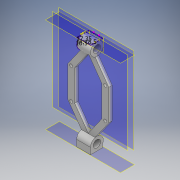
# Autodesk Inventor part: mousetrapMount
Saved by Autodesk Inventor 2018 (Build 220112000, 112)
## iProperties
Created: 2018-11-24
Part Number: mousetrapMount
Material: Generic
Document SubType Name: Modeling
Designer: Prakash
Density: 1 g/cm^3
Appearance: Default
Author: Prakash
Autodesk Inventor part; units mm, degrees
ref_plane "YZ Plane" through (0, 0, 0) normal (1, 0, 0) x (0, 1, 0)
ref_plane "XY Plane" through (0, 0, 0) normal (0, 0, 1) x (1, 0, 0)
sketch "Sketch3" plane through (0, 0, 0) normal (1, 0, 0) x (0, 1, 0)
  circle A0 centre (0, 0) radius 5.25
  circle A1 centre (0, 0) radius 9.25
  dimension "d0" = 10.5
  dimension "d1" = 18.5
  constraints: 2 centre point, 2 coincident
  measures "d0" diameter of A0
  measures "d1" diameter of A1
extrude "Extrusion1" add sketch "Sketch3" along normal blind 20
ref_plane "Work Plane1" through (0, 9.25, 0) normal (0, 1, 0) x (-1, 0, 0)
sketch "Sketch4" plane through (0, 9.25, 0) normal (0, 1, 0) x (-1, 0, 0)
  line L0 (-20, 9.25) -> (-20, -9.25) projected
  line L1 (-20, 0) -> (0, 0) construction
  line L2 (0, 9.25) -> (-20, 9.25) projected
  line L3 (-20, 9.25) -> (-20, -9.25) projected
  line L4 (0, -9.25) -> (0, 9.25) projected
  line L5 (0, -9.25) -> (-20, -9.25) construction
  line L6 (-59.213, -14.8) -> (39.213, -14.8) construction
  line L7 (39.213, -14.8) -> (39.213, -59.25) construction
  line L8 (39.213, -59.25) -> (-59.213, -59.25) construction
  line L9 (-59.213, -59.25) -> (-59.213, -14.8) construction
  line L10 (-59.213, -14.8) -> (39.213, -59.25) construction
  line L11 (39.213, -14.8) -> (-59.213, -59.25) construction
  line L12 (-59.213, -59.25) -> (39.213, -59.25) construction
  line L13 (39.213, -59.25) -> (39.213, -103.7) construction
  line L14 (39.213, -103.7) -> (-59.213, -103.7) construction
  line L15 (-59.213, -103.7) -> (-59.213, -59.25) construction
  line L16 (-59.213, -59.25) -> (39.213, -103.7) construction
  line L17 (39.213, -59.25) -> (-59.213, -103.7) construction
  line L18 (-10, -37.025) -> (-59.213, -37.025) construction
  line L19 (-10, -37.025) -> (39.213, -37.025) construction
  line L20 (-10, -81.475) -> (-59.213, -81.475) construction
  line L21 (-10, -81.475) -> (39.213, -81.475) construction
  line L22 (-20, -9.25) -> (-39.6065, -37.025)
  line L23 (-10, -9.25) -> (-29.6065, -37.025)
  line L24 (-39.6065, -37.025) -> (-39.6065, -59.25)
  line L25 (-10, -9.25) -> (9.6065, -37.025)
  line L26 (0, -9.25) -> (19.6065, -37.025)
  line L27 (19.6065, -37.025) -> (19.6065, -59.25)
  line L28 (-34.6065, -37.025) -> (-34.6065, -81.475) construction
  line L29 (14.6065, -81.475) -> (14.6065, -37.025) construction
  line L30 (-29.6065, -37.025) -> (-29.6065, -59.25)
  line L31 (9.6065, -37.025) -> (9.6065, -59.25)
  line L32 (-39.6065, -59.25) -> (-29.6065, -59.25)
  line L33 (9.6065, -59.25) -> (19.6065, -59.25)
  line L34 (-20, -9.25) -> (-10, -9.25)
  line L35 (0, -9.25) -> (-20, -9.25) projected
  line L36 (-10, -9.25) -> (0, -9.25)
  point P0 (-10, 0)
  dimension "d5" = 44.45
  dimension "d6" = 49.213
  dimension "d7" = 44.45
  dimension "d21" = 50
  constraints: 62 end point, 15 midpoint, 10 point on line, 8 parallel, 5 perpendicular, 3 horizontal, 2 collinear, 2 vertical, 1 equal length, 2 other
  measures "d5" distance of L6.end L7.end
  measures "d6" distance from line of L7 L18.start
  measures "d7" distance of L12.end L13.end
  measures "d21" distance between parallel lines of L8 L5
ref_plane "Work Plane2" through (0, 0, 0) normal (0, 1, 0) x (-1, 0, 0)
sketch "Sketch5" plane through (0, 0, 0) normal (0, 1, 0) x (-1, 0, 0)
  line L0 (-20, -9.25) -> (-39.6065, -37.025) projected
  line L1 (-10, -9.25) -> (-29.6065, -37.025) projected
  line L2 (-10, -9.25) -> (9.6065, -37.025) projected
  line L3 (0, -9.25) -> (19.6065, -37.025) projected
  line L4 (19.6065, -37.025) -> (19.6065, -59.25) projected
  line L5 (9.6065, -37.025) -> (9.6065, -59.25) projected
  line L6 (-29.6065, -37.025) -> (-29.6065, -59.25) projected
  line L7 (-39.6065, -37.025) -> (-39.6065, -59.25) projected
  line L8 (-39.6065, -59.25) -> (-29.6065, -59.25) projected
  line L9 (9.6065, -59.25) -> (19.6065, -59.25) projected
  line L10 (0, -9.25) -> (-20, -9.25) projected
  point P0 (0, 0)
  point P1 (-34.6065, -37.025)
  point P2 (14.6065, -37.025)
extrude "Extrusion2" add sketch "Sketch5" along normal mid plane 5
sketch "Sketch7" plane through (0, -2.5, 0) normal (0, -1, 0) x (1, 0, 0)
  point P0 (0, 0)
  point P1 (34.6065, -37.025)
  point P2 (-14.6065, -37.025)
hole "Hole1" at (-14.6065, -2.5, -37.025) at (34.6065, -2.5, -37.025) direction (0, 1, 0) diameter 4.305 end through all clearance for "Flat Head Machine Screw (82)" size "#6" standard "Ansi Unified Screw Threads"
sketch "Sketch8" plane through (0, 0, -9.25) normal (0, 0, 1) x (-1, 0, 0)
  line L0 (0, -2.5) -> (-10, -2.5) projected
  line L1 (-20, 0) -> (-20, 2.5) projected
  line L2 (0, -2.5) -> (-20, -2.5)
  line L3 (-20, -2.5) -> (-20, 2.5)
  line L4 (-20, 2.5) -> (0, 2.5)
  line L5 (0, 2.5) -> (0, -2.5)
  point P0 (0, 0)
  constraints: 8 end point, 2 parallel, 1 horizontal, 1 perpendicular
extrude "Extrusion4" add sketch "Sketch8" along normal up to surface round surface about axis through (0, 0, 0) along (1, 0, 0) radius 9.25 far side no
ref_plane "Work Plane3" through (0, 0, 9.25) normal (0, 0, -1) x (-1, 0, 0)
ref_plane "Work Plane4" through (0, 0, -127.75) normal (0, 0, -1) x (-1, 0, 0)
ref_plane "Work Plane5" through (0, 9.25, 0) normal (0, 1, 0) x (-1, 0, 0)
sketch "Sketch14" plane through (0, 9.25, 0) normal (0, 1, 0) x (-1, 0, 0)
  line L0 (-20, -8.9058) -> (0, -8.9058) projected
  line L1 (0, -8.9058) -> (0, -8.9058) projected
  line L2 (0, -8.9058) -> (-20, -8.9058) projected
  line L3 (-20, -8.9058) -> (-20, -8.9058) projected
  line L4 (-20, 9.25) -> (-20, -8.9058) projected
  line L5 (0, -8.9058) -> (0, 9.25) projected
  line L6 (-20, -8.9058) -> (0, 9.25) construction
  line L7 (-20, 9.25) -> (0, -8.9058) construction
  point P0 (0, 0)
  point P1 (-10, 0.1721)
  constraints: 4 end point, 1 midpoint
sketch "Sketch15" plane through (0, 9.25, 0) normal (0, 1, 0) x (-1, 0, 0)
  line L0 (-20, 9.25) -> (0, -8.9058) construction
  line L1 (-20, -8.9058) -> (0, 9.25) construction
  circle A0 centre (-10, 0.1721) radius 4
  point P0 (0, 0)
  dimension "d28" = 8
  constraints: 1 centre point, 1 coincident
  measures "d28" diameter of A0
extrude "Extrusion6" add sketch "Sketch15" against normal up to surface round surface about axis through (0, 0, 0) along (1, 0, 0) radius 9.25 far side no
extrude "Extrusion7" add sketch "Sketch15" along normal blind 1
sketch "Sketch16" plane through (10, 10.25, 0.1721) normal (0, 1, 0) x (1, 0, 0)
  line L0 (10, 9.0779) -> (-10, -9.0779) construction
  line L1 (10, -9.0779) -> (-10, 9.0779) construction
  circle A0 centre (0, 0) radius 4 projected
  circle A1 centre (0, 0) radius 2.5275
  point P0 (-10, 0.1721)
  dimension "d33" = 5.055
  constraints: 1 centre point, 1 coincident
  measures "d33" diameter of A1
extrude "Extrusion8" cut sketch "Sketch16" against normal blind 3.81 contours A1
sketch "Sketch17" plane through (10, 10.25, 0.1721) normal (0, 1, 0) x (1, 0, 0)
  line L0 (10, -9.0779) -> (-10, 9.0779) construction
  line L1 (10, 9.0779) -> (-10, -9.0779) construction
  circle A0 centre (0, 0) radius 2.6545
  point P0 (-10, 0.1721)
  dimension "d36" = 5.309
  constraints: 1 centre point, 1 coincident
  measures "d36" diameter of A0
loft "Loft1" cut profiles "Sketch17" section 1 edges at (7.4725, 6.44, 0.1721)
sketch "Sketch18" plane through (10, 6.44, 0.1721) normal (0, 1, 0) x (1, 0, 0)
  line L0 (10, -9.0779) -> (-10, 9.0779) construction
  line L1 (10, 9.0779) -> (-10, -9.0779) construction
  circle A0 centre (0, 0) radius 1.8
  point P0 (-10, 0.1721)
  dimension "d41" = 3.6
  constraints: 1 centre point, 1 coincident
  measures "d41" diameter of A0
extrude "Extrusion9" cut sketch "Sketch18" against normal up to surface round surface about axis through (0, 0, 0) along (1, 0, 0) radius 5.25 far side no
mirror "Mirror3" about plane through (39.6065, 0, -59.25) normal (0, 0, -1) of "Extrusion1", "Extrusion2", "Hole1", "Extrusion4", "Extrusion6", "Extrusion7", "Extrusion8", "Loft1", "Extrusion9"
sketch "Sketch21" plane through (0, 0, 9.25) normal (0, 0, -1) x (-1, 0, 0)
  line L0 (-20, 9.25) -> (-20, -9.25) construction
  line L1 (0, -9.25) -> (0, 9.25) construction
  line L2 (0, -9.25) -> (-20, -9.25) construction
  line L3 (0, -9.25) -> (-20, -9.25)
  line L4 (-20, -9.25) -> (-20, 8.1)
  line L5 (-20, 8.1) -> (0, 8.1)
  line L6 (0, 8.1) -> (0, -9.25)
  point P0 (0, 0)
  point P1 (-20, 2.5)
  point P2 (-20, -2.5)
  point P3 (0, -2.5)
  point P4 (0, 2.5)
  dimension "d45" = 17.35
  constraints: 8 end point, 2 perpendicular, 2 point on line, 1 horizontal, 1 horizontal alignment
  measures "d45" distance between parallel lines of L2 L5
sketch "Sketch22" plane through (0, 0, -127.75) normal (0, 0, -1) x (-1, 0, 0)
  line L0 (0, -9.25) -> (-20, -9.25) construction
  line L1 (-20, 9.25) -> (-20, -9.25) construction
  line L2 (-20, 8.1) -> (0, 8.1) projected
  line L3 (0, -9.25) -> (0, 9.25) construction
  line L4 (-20, 8.1) -> (-20, -9.25)
  line L5 (0, -9.25) -> (-20, -9.25)
  line L6 (0, -9.25) -> (0, 8.1)
  point P0 (0, 0)
  constraints: 6 end point, 2 perpendicular, 1 vertical
extrude "Extrusion10" add sketch "Sketch22" against normal up to surface round surface about axis through (0, 0, -118.5) along (-1, 0, 0) radius 9.25 far side no
equation "\"d7\" = d5"
body "Solid1"
